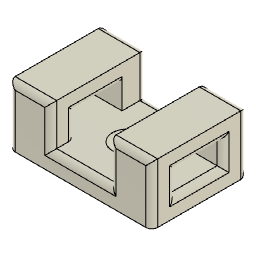
cable_anchor (Autodesk Fusion 360 design; units mm, degrees)
Autodesk Fusion 360 part; units mm, degrees
sketch "Sketch1" plane through (0, 0, 0) normal (0, 0, 1) x (1, 0, 0)
  line L0 (-5, 5) -> (5, 5)
  line L1 (5, 5) -> (5, -5)
  line L2 (5, -5) -> (-5, -5)
  line L3 (-5, -5) -> (-5, 5)
  dimension "d1" = 10
  dimension "d2" = 10
  constraint horizontal L0
  constraint vertical L1
  constraint horizontal L2
  constraint vertical L3
  measures "d1" distance of L0.start L0.end
  measures "d2" distance of L0.start L2.end
extrude "Extrude1" add sketch "Sketch1" along normal blind 2 makes body 1
sketch "Sketch2" plane through (0, 0, 2) normal (0, 0, 1) x (-1, 0, 0)
  line L0 (5, 5) -> (-5, 5)
  line L1 (-5, 5) -> (-5, -5)
  line L2 (-5, -5) -> (5, -5)
  line L3 (5, -5) -> (5, 5)
  line L4 (5, -5) -> (3, -5)
  line L5 (3, -5) -> (3, -3)
  line L6 (3, -3) -> (5, -3)
  line L7 (5, -3) -> (5, -5)
  line L8 (-3, -5) -> (-5, -5)
  line L9 (-5, -5) -> (-5, -3)
  line L10 (-5, -3) -> (-3, -3)
  line L11 (-3, -3) -> (-3, -5)
  line L12 (5, 3) -> (3, 3)
  line L13 (3, 3) -> (3, 5)
  line L14 (3, 5) -> (5, 5)
  line L15 (5, 5) -> (5, 3)
  line L16 (-3, 3) -> (-5, 3)
  line L17 (-5, 3) -> (-5, 5)
  line L18 (-5, 5) -> (-3, 5)
  line L19 (-3, 5) -> (-3, 3)
  line L20 (5, -5) -> (3, -5)
  line L21 (3, -5) -> (3, 5)
  line L22 (3, 5) -> (5, 5)
  line L23 (5, 5) -> (5, -5)
  line L24 (3, -5) -> (-3, -5)
  line L25 (-3, -5) -> (-3, -3)
  line L26 (-3, -3) -> (3, -3)
  line L27 (3, -3) -> (3, -5)
  line L28 (-3, -3) -> (-5, -3)
  line L29 (-5, -3) -> (-5, 3)
  line L30 (-5, 3) -> (-3, 3)
  line L31 (-3, 3) -> (-3, -3)
  line L32 (-3, 3) -> (3, 3)
  line L33 (3, 3) -> (3, 5)
  line L34 (3, 5) -> (-3, 5)
  line L35 (-3, 5) -> (-3, 3)
  constraint horizontal L4
  constraint vertical L5
  constraint horizontal L6
  constraint vertical L7
  constraint coincident L2.end L3.start
  constraint horizontal L8
  constraint vertical L9
  constraint horizontal L10
  constraint vertical L11
  constraint coincident L1 L9.end
  constraint coincident L2 L8.start
  constraint horizontal L12
  constraint vertical L13
  constraint horizontal L14
  constraint vertical L15
  constraint coincident L0 L13.end
  constraint coincident L3 L12.start
  constraint horizontal L16
  constraint vertical L17
  constraint horizontal L18
  constraint vertical L19
  constraint coincident L0.end L1.start
  constraint horizontal L20
  constraint vertical L21
  constraint horizontal L22
  constraint vertical L23
  constraint horizontal L24
  constraint vertical L25
  constraint horizontal L26
  constraint vertical L27
  constraint horizontal L28
  constraint vertical L29
  constraint horizontal L30
  constraint vertical L31
  constraint horizontal L32
  constraint vertical L33
  constraint horizontal L34
  constraint vertical L35
extrude "Extrude2" add sketch "Sketch2" along normal blind 2 contours L0 L3 L12 L13 L14 L15 L21 L22 L23 L33 | L0 L1 L16 L17 L18 L19 L30 L35 | L2 L3 L4 L5 L6 L7 L20 L21 L23 L27 | L1 L2 L8 L9 L10 L11 L25 L28 bodies 1
sketch "Sketch3" plane through (0, 0, 2) normal (0, 0, 1) x (-1, 0, 0)
  line L0 (5, 3) -> (3, 3)
  line L1 (3, 3) -> (3, 5)
  line L2 (3, 5) -> (-3, 5)
  line L3 (-3, 5) -> (-3, 3)
  line L4 (-3, 3) -> (-5, 3)
  line L5 (-5, 3) -> (-5, -3)
  line L6 (-5, -3) -> (-3, -3)
  line L7 (-3, -3) -> (-3, -5)
  line L8 (-3, -5) -> (3, -5)
  line L9 (3, -5) -> (3, -3)
  line L10 (3, -3) -> (5, -3)
  line L11 (5, -3) -> (5, 3)
  line L12 (5, -3) -> (3, -3)
  line L13 (3, -3) -> (3, 3)
  line L14 (3, 3) -> (5, 3)
  line L15 (5, 3) -> (5, -3)
  line L16 (-3, -3) -> (-5, -3)
  line L17 (-5, -3) -> (-5, 3)
  line L18 (-5, 3) -> (-3, 3)
  line L19 (-3, 3) -> (-3, -3)
  constraint horizontal L12
  constraint vertical L13
  constraint horizontal L14
  constraint vertical L15
  constraint coincident L0.end L1.start
  constraint coincident L10.end L11.start
  constraint horizontal L16
  constraint vertical L17
  constraint horizontal L18
  constraint vertical L19
  constraint coincident L4.end L5.start
  constraint coincident L6.end L7.start
extrude "Extrude3" add sketch "Sketch3" along normal blind 4 and the other way blind -2 separate body contours L0 L10 L11 L12 L13 L14 L15 | L4 L5 L6 L16 L17 L18 L19 makes body 2 at (-3.6667, -1, 4) makes body 3 at (4.3333, -1, 4)
extrude "Extrude4" add 4 faces at (-3.6667, -4.3333, 4) (4.3333, -4.3333, 4) (-3.6667, 3.6667, 4) (4.3333, 3.6667, 4) along direction (0, 0, 1) blind 2 on bodies 1 bodies 1 2 3
extrude "Extrude5" add 1 faces at (5, 1, 5.3333) along direction (1, 0, 0) blind 1 on bodies 1 bodies 1
extrude "Extrude6" add 1 faces at (-5, 1, 5.3333) along direction (-1, 0, 0) blind 1 on bodies 1 bodies 1
sketch "Sketch5" plane through (0, 0, 0) normal (1, 0, 0) x (0, 1, 0)
sketch "Sketch6" plane through (0, 0, 2) normal (0, 0, 1) x (-1, 0, 0)
  line L0 (6, 3) -> (3, 3)
  line L1 (-3, 3) -> (-6, 3)
  line L2 (-6, -3) -> (-3, -3)
  line L3 (3, -3) -> (6, -3)
  circle A0 centre (0, 0) radius 1.625
  line L4 (3, 3) -> (3, 5)
  line L5 (3, 5) -> (-3, 5)
  line L6 (-3, 5) -> (-3, 3)
  line L7 (-6, 3) -> (-6, -3)
  line L8 (-3, -3) -> (-3, -5)
  line L9 (-3, -5) -> (3, -5)
  line L10 (3, -5) -> (3, -3)
  line L11 (6, -3) -> (6, 3)
  dimension "d35" = 3.25
  constraint coincident A0.centre origin
  measures "d35" diameter of A0
extrude "Extrude7" cut sketch "Sketch6" against normal blind 2 contours A0 bodies 1
extrude "Extrude8" add 1 faces at (-5, -5, 2.6667) along direction (0, -1, 0) blind 2 on bodies 1 bodies 1
extrude "Extrude9" add 1 faces at (-6, -5.6667, 3.3333) along direction (-1, 0, 0) blind 2 on bodies 1 bodies 1
extrude "Extrude10" add 1 faces at (-6.3333, 5, 2.6667) along direction (0, 1, 0) blind 2 on bodies 1 bodies 1
extrude "Extrude11" add 1 faces at (6, 5.6667, 2.6667) along direction (1, 0, 0) blind 2 on bodies 1 bodies 1
extrude "Extrude12" add 2 faces at (4.6667, 2.3333, 6) (-6.3333, -2.3333, 6) along direction (0, 0, 1) blind 2 on bodies 1 bodies 1
extrude "Extrude13" cut 1 faces at (4.6667, -1, 4) along direction (0, 0, 1) blind 2 on bodies 1 bodies 1
extrude "Extrude14" cut 1 faces at (4.6667, -3, 3.3333) along direction (0, -1, 0) blind 1 on bodies 1 bodies 1
extrude "Extrude15" cut 1 faces at (6.3333, 3, 4.6667) along direction (0, 1, 0) blind 1 on bodies 1 bodies 1
extrude "Extrude16" cut 1 faces at (-6.3333, 3, 3.3333) along direction (0, 1, 0) blind 1 on bodies 1 bodies 1
extrude "Extrude17" cut 1 faces at (-6.3333, -3, 3.3333) along direction (0, -1, 0) blind 1 on bodies 1 bodies 1
extrude "Extrude18" cut 1 faces at (-4.6667, -1.3333, 4) along direction (0, 0, 1) blind 1 on bodies 1 bodies 1
extrude "Extrude19" add 1 faces at (4.6667, 2.3333, 8) along direction (0, 0, 1) blind 1 on bodies 1 bodies 1
extrude "Extrude20" add 1 faces at (-8, 1.3333, 7) along direction (-1, 0, 0) blind 1 on bodies 1 bodies 1
extrude "Extrude21" add 1 faces at (-5, 2.3333, 8) along direction (0, 0, 1) blind 1 on bodies 1 bodies 1
extrude "Extrude22" cut 1 faces at (-7, -1.3333, 5) along direction (0, 0, 1) blind 1 on bodies 1 bodies 1
extrude "Extrude23" add 1 faces at (-6.5417, 0, 0) along direction (0, 0, -1) blind 1 on bodies 1 bodies 1
extrude "Extrude24" add 1 faces at (-9, 1.3333, 0) along direction (-1, 0, 0) blind 1 on bodies 1 bodies 1
extrude "Extrude25" add 1 faces at (8, 1.3333, 0) along direction (1, 0, 0) blind 1 on bodies 1 bodies 1
extrude "Extrude26" add 1 faces at (-7.6667, -7, 3.3333) along direction (0, -1, 0) blind 1 on bodies 1 bodies 1
extrude "Extrude27" add 1 faces at (-7.6667, 7, 3.3333) along direction (0, 1, 0) blind 1 on bodies 1 bodies 1
extrude "Extrude28" cut 1 faces at (-3, 6.6667, 5.6667) along direction (-1, 0, 0) blind 1 on bodies 1 bodies 1
extrude "Extrude29" cut 1 faces at (3, 6.6667, 5.6667) along direction (1, 0, 0) blind 1 on bodies 1 bodies 1
extrude "Extrude30" cut 1 faces at (4, 6.6667, 5.6667) along direction (1, 0, 0) blind 1 on bodies 1 bodies 1
extrude "Extrude31" cut 1 faces at (-4, 6.6667, 5.6667) along direction (-1, 0, 0) blind 1 on bodies 1 bodies 1
extrude "Extrude32" add 1 faces at (9, 6.6667, 3.3333) along direction (1, 0, 0) blind 2 on bodies 1 bodies 1
extrude "Extrude33" add 1 faces at (-10, 6.6667, 3.3333) along direction (-1, 0, 0) blind 2 on bodies 1 bodies 1
extrude "Extrude34" add 1 faces at (11, 6.6667, 3.3333) along direction (1, 0, 0) blind 1 on bodies 1 bodies 1
fillet "Fillet10" radius 1 7 edges at (12, -8, 4) (8.5, -8, 9) (5, -8, 5.5) (0, -8, 2) (-5, -8, 5.5) (-8.5, -8, 9) (-12, -8, 4) on bodies 1
fillet "Fillet11" radius 1 6 edges at (-5, 8, 5.5) (-8.5, 8, 9) (-12, 8, 4) (0, 8, 2) (5, 8, 5.5) (8.5, 8, 9) 1 faces at (9.6667, 8, 3.3333) on bodies 1
fillet "Fillet12" radius 1 4 edges at (-12, 0, 6) (-12, 4, 4) (-12, 0, 2) (-12, -4, 4) on bodies 1
fillet "Fillet13" radius 1 6 edges at (12, 0, 6) (-5, 0, 6) (-5, -4, 4) (12, -4, 4) (12, 0, 2) (12, 4, 4) on bodies 1
fillet "Fillet14" radius 1 3 edges at (5, 4, 4) (5, 0, 6) (5, -4, 4) on bodies 1
fillet "Fillet15" radius 1 1 edges at (1.515, -0.5876, 2) on bodies 1
